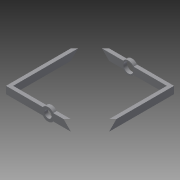
# Autodesk Inventor part: joystick_mount
Saved by Autodesk Inventor 2015 (Build 190159000, 159)
## iProperties
Created: 2015-12-08
Part Number: joystick_mount
Material: Generic
Document SubType Name: Modeling
Designer: boztalay
Density: 1 g/cm^3
Appearance: Default
Author: boztalay
Autodesk Inventor part; units mm, degrees
ref_plane "YZ Plane" through (0, 0, 0) normal (1, 0, 0) x (0, 1, 0)
ref_plane "XZ Plane" through (0, 0, 0) normal (0, 1, 0) x (-1, 0, 0)
ref_plane "XY Plane" through (0, 0, 0) normal (0, 0, 1) x (1, 0, 0)
sketch "Sketch1" plane through (0, 0, 0) normal (0, 1, 0) x (-1, 0, 0)
  line L0 (-67.31, 67.31) -> (67.31, 67.31)
  line L1 (67.31, 67.31) -> (67.31, -67.31)
  line L2 (67.31, -67.31) -> (-67.31, -67.31)
  line L3 (-67.31, -67.31) -> (-67.31, 67.31)
  line L4 (-67.31, 67.31) -> (67.31, -67.31) construction
  line L5 (67.31, 67.31) -> (-67.31, -67.31) construction
  line L6 (-73.66, 73.66) -> (73.66, 73.66)
  line L7 (73.66, 73.66) -> (73.66, -73.66)
  line L8 (73.66, -73.66) -> (-73.66, -73.66)
  line L9 (-73.66, -73.66) -> (-73.66, 73.66)
  line L10 (-73.66, 73.66) -> (73.66, -73.66) construction
  line L11 (73.66, 73.66) -> (-73.66, -73.66) construction
  point P0 (0, 0)
  dimension "d0" = 134.62
  dimension "d1" = 134.62
  dimension "d2" = 147.32
  dimension "d3" = 147.32
  constraints: 24 end point, 4 midpoint, 4 parallel, 2 horizontal, 2 perpendicular
  measures "d0" distance of L0.end L1.end
  measures "d1" distance of L1.end L2.end
  measures "d2" distance of L7.end L8.end
  measures "d3" distance of L6.end L7.end
extrude "Extrusion1" add sketch "Sketch1" along normal blind 12.7
sketch "Sketch2" plane through (73.66, 0, -73.66) normal (0, 0, -1) x (-1, 0, 0)
  circle A0 centre (73.66, 6.35) radius 11.1125
  point P0 (73.66, 0)
  dimension "d6" = 22.225
  constraints: 1 centre point
  measures "d6" diameter of A0
extrude "Extrusion2" add sketch "Sketch2" against normal up to surface (6.35 mm away)
sketch "Sketch3" plane through (73.66, 0, -73.66) normal (0, 0, -1) x (-1, 0, 0)
  circle A0 centre (73.66, 6.35) radius 8.7313
  point P0 (73.66, 0)
  dimension "d9" = 17.4625
  constraints: 1 centre point
  measures "d9" diameter of A0
extrude "Extrusion3" cut sketch "Sketch3" against normal up to next
sketch "Sketch4" plane through (-73.66, 0, 73.66) normal (0, 0, 1) x (1, 0, 0)
  circle A0 centre (73.66, 6.35) radius 11.1125
  point P0 (73.66, 0)
  dimension "d12" = 22.225
  constraints: 1 centre point
  measures "d12" diameter of A0
extrude "Extrusion4" add sketch "Sketch4" against normal up to surface (6.35 mm away)
sketch "Sketch5" plane through (-73.66, 0, 73.66) normal (0, 0, 1) x (1, 0, 0)
  circle A0 centre (73.66, 6.35) radius 6.35
  point P0 (73.66, 0)
  dimension "d15" = 12.7
  constraints: 1 centre point
  measures "d15" diameter of A0
extrude "Extrusion5" cut sketch "Sketch5" against normal up to next
body "Solid1"
